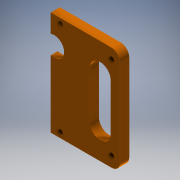
# Autodesk Inventor part: Carro XY_trava_B
Saved by Autodesk Inventor 2016 (Build 200138000, 138)
## iProperties
Created: 2016-08-11
Part Number: Carro XY_trava_B
Material: ABS Plastic
Document SubType Name: Modeling
Designer: Waldo
Density: 1.06 g/cm^3
Appearance: Smooth - White
Author: Waldo
Autodesk Inventor part; units mm, degrees
ref_plane "YZ Plane" through (0, 0, 0) normal (1, 0, 0) x (0, 1, 0)
ref_plane "XZ Plane" through (0, 0, 0) normal (0, 1, 0) x (-1, 0, 0)
sketch "Sketch1" plane through (0, 0, 0) normal (0, 1, 0) x (-1, 0, 0)
  line L0 (4.4839, 27.6452) -> (-35.5161, 27.6452)
  line L1 (-35.5161, 27.6452) -> (-35.5161, -32.3548)
  line L2 (-35.5161, -32.3548) -> (4.4839, -32.3548)
  line L3 (4.4839, -32.3548) -> (4.4839, 27.6452)
  point P0 (0, 0)
  dimension "d0" = 60
  dimension "d1" = 40
  constraints: 8 end point, 2 parallel, 1 horizontal, 1 perpendicular
  measures "d0" distance of L2.end L0.start
  measures "d1" distance of L0.start L0.end
extrude "Extrusion1" add sketch "Sketch1" along normal blind 5.2
fillet "Fillet1" radius 5 2 edges at (35.5161, 2.6, -32.3548) (35.5161, 2.6, 27.6452)
sketch "Sketch2" plane through (0, 0, 0) normal (0, -1, 0) x (1, 0, 0)
  circle A0 centre (30.5161, 21.6452) radius 1.5 projected
  circle A1 centre (1.0161, 24.6452) radius 1.5 projected
  circle A2 centre (1.0161, -29.3548) radius 1.5 projected
  circle A3 centre (30.5161, -26.3548) radius 1.5 projected
  point P0 (0, 0)
  constraints: 4 coincident
hole "Hole1" at (30.5161, 0, 21.6452) at (30.5161, 0, -26.3548) at (1.0161, 0, -29.3548) at (1.0161, 0, 24.6452) direction (0, 1, 0) diameter 3 end through all
sketch "Sketch3" plane through (0, 5.2, 0) normal (0, 1, 0) x (1, 0, 0)
  circle A0 centre (-2.4839, -11.6452) radius 7.9 projected
  point P0 (0, 0)
ref_plane "Work Plane1" through (-10.3839, 4.1, 4.0025) normal (0, 1, 0) x (0, 0, 1)
extrude "Extrusion2" cut sketch "Sketch3" against normal up to surface (1.1 mm away)
sketch "Sketch4" plane through (-2.4839, 4.1, 11.6452) normal (0, 1, 0) x (1, 0, 0)
  arc A0 (-2, 5.3376) -> (-2, -5.3376) centre (0, 0) ccw projected
  circle A1 centre (0, 0) radius 5.5 projected
  circle A2 centre (0, 0) radius 5.7
  point P0 (2.4839, 11.6452)
  dimension "d14" = 11.4
  constraints: 1 centre point
  measures "d14" diameter of A2
extrude "Extrusion3" cut sketch "Sketch4" against normal through all contours A2 A0 | A1
sketch "Sketch5" plane through (0, 0, 0) normal (0, -1, 0) x (1, 0, 0)
  circle A0 centre (24.0161, 11.1452) radius 6 projected
  circle A1 centre (24.0161, -15.8548) radius 6 projected
  line L0 (24.0161, 11.1452) -> (24.0161, -15.8548) construction
  line L1 (18.0161, 11.1452) -> (18.0161, -15.8548)
  line L2 (30.0161, -15.8548) -> (30.0161, 11.1452)
  arc A2 (30.0161, 11.1452) -> (18.0161, 11.1452) centre (24.0161, 11.1452) ccw
  arc A3 (18.0161, -15.8548) -> (30.0161, -15.8548) centre (24.0161, -15.8548) ccw
  point P0 (0, 0)
  point P1 (24.0161, -2.3548)
  constraints: 8 end point, 4 point on circle, 4 tangent, 2 centre point, 1 concentric, 1 midpoint, 1 parallel, 1 vertical
extrude "Extrusion4" cut sketch "Sketch5" against normal through all
body "Solid1"
